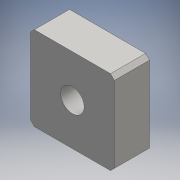
# Autodesk Inventor part: GearHead1
Saved by Autodesk Inventor 2016 (Build 200138000, 138)
## iProperties
Created: 2016-06-23
Part Number: GearHead1
Material: 一般
Document SubType Name: Modeling
Designer: 宏太
Density: 1 g/cm^3
Appearance: 既定
Mass: 31.1022 g
Surface Area: 71.4604 cm^2
Volume: 31.1022 cm^3
Author: 宏太
Autodesk Inventor part; units mm, degrees
ref_plane "YZ Plane" through (0, 0, 0) normal (1, 0, 0) x (0, 1, 0)
ref_plane "XZ Plane" through (0, 0, 0) normal (0, 1, 0) x (-1, 0, 0)
ref_plane "XY Plane" through (0, 0, 0) normal (0, 0, 1) x (1, 0, 0)
sketch "スケッチ1" plane through (0, 0, 0) normal (0, 1, 0) x (-1, 0, 0)
  line L0 (-21.5, -21.5) -> (21.5, -21.5)
  line L1 (21.5, -21.5) -> (21.5, 21.5)
  line L2 (21.5, 21.5) -> (-21.5, 21.5)
  line L3 (-21.5, 21.5) -> (-21.5, -21.5)
  line L4 (-21.5, -21.5) -> (21.5, 21.5) construction
  line L5 (21.5, -21.5) -> (-21.5, 21.5) construction
  point P0 (0, 0)
  dimension "d0" = 43
  dimension "d1" = 43
  constraints: 12 end point, 2 midpoint, 2 parallel, 1 horizontal, 1 perpendicular
  measures "d0" distance of L2.end L1.end
  measures "d1" distance of L1.end L0.end
extrude "押し出し1" add sketch "スケッチ1" along normal blind 18
chamfer "面取り1" distance 2 angle 45 1 edges at (21.5, 9, 21.5)
chamfer "面取り2" distance 2 angle 45 1 edges at (21.5, 9, -21.5)
chamfer "面取り3" distance 2 angle 45 1 edges at (-21.5, 9, 21.5)
chamfer "面取り4" distance 2 angle 45 1 edges at (-21.5, 9, -21.5)
sketch "スケッチ2" plane through (0, 0, 0) normal (0, 1, 0) x (-1, 0, 0)
  circle A0 centre (0, 0) radius 6
  dimension "d16" = 12
  constraints: 1 centre point, 1 coincident
  measures "d16" diameter of A0
extrude "押し出し2" cut sketch "スケッチ2" along normal blind 18
